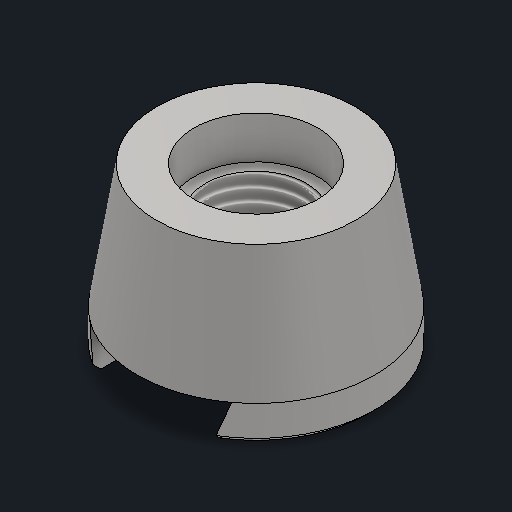
# Autodesk Inventor part: 0.375 Shaft Dovetail
Saved by Autodesk Inventor 2025.1 (Build 291241020, 241B)
## iProperties
Created: 2025-05-15
Part Number: 0.375 Shaft Dovetail
Material: Stainless Steel
Document SubType Name: Modeling
Designer: Joshua Eah
Density: 8 g/cm^3
Appearance: Semi-Polished
Author: Joshua Eah
Autodesk Inventor part; units mm, degrees
ref_plane "YZ Plane" through (0, 0, 0) normal (1, 0, 0) x (0, 1, 0)
sketch "Sketch1" plane through (0, 0, 0) normal (0, 1, 0) x (-1, 0, 0)
  circle A0 centre (0, 0) radius 4.9911
  dimension "d0" = 9.9822
  constraints: 1 centre point, 1 coincident
  measures "d0" diameter of A0
extrude "Extrusion1" add sketch "Sketch1" along normal blind 1.524
sketch "Sketch2" plane through (0, 1.524, 0) normal (0, 1, 0) x (1, 0, 0)
  point P0 (0, 0)
ref_plane "Work Plane1" through (0, 6.731, 0) normal (0, -1, 0) x (1, 0, 0)
sketch "Sketch3" plane through (0, 6.731, 0) normal (0, -1, 0) x (1, 0, 0)
  circle A0 centre (0, 0) radius 4.1593
  circle A1 centre (0, 0) radius 2.6035
  dimension "d4" = 8.3185
  dimension "d9" = 5.207
  constraints: 2 centre point, 2 coincident
  measures "d4" diameter of A0
  measures "d9" diameter of A1
loft "Loft1" add profiles "Sketch3" section 1 edges at (4.9911, 1.524, 0) contours A0 | A1
hole "Hole1" at (0, 6.731, 0) direction (0, -1, 0) diameter 4.2418 end through all thread size "10-48 UNS" class "2B" standard "ANSI Unified Screw Threads"
extrude "Extrusion3" cut sketch "Sketch3" along normal blind 1.778 contours A1
ref_plane "Work Plane2" through (0, 0, -4.9911) normal (0, 0, 1) x (1, 0, 0)
chamfer "Chamfer1" distance 0.254 angle 45 1 edges at (4.9911, 0, 0)
sketch "Sketch4" plane through (0, 0, -4.9911) normal (0, 0, 1) x (1, 0, 0)
  line L0 (4.9911, 1.524) -> (-4.9911, 1.524) projected
  line L1 (0, 1.524) -> (0, 0)
  line L2 (2.5082, 1.524) -> (-2.5083, 1.524)
  line L3 (-2.5083, 1.524) -> (-2.5083, 0)
  line L4 (-2.5083, 0) -> (2.5082, 0)
  line L5 (2.5082, 0) -> (2.5082, 1.524)
  line L6 (2.5082, 1.524) -> (-2.5083, 0) construction
  line L7 (-2.5083, 1.524) -> (2.5082, 0) construction
  line L8 (2.9845, 1.524) -> (-2.9845, 1.524)
  line L9 (-2.9845, 1.524) -> (-2.9845, 0)
  line L10 (-2.9845, 0) -> (2.9845, 0)
  line L11 (2.9845, 0) -> (2.9845, 1.524)
  line L12 (2.9845, 1.524) -> (-2.9845, 0) construction
  line L13 (-2.9845, 1.524) -> (2.9845, 0) construction
  line L14 (2.9845, 1.524) -> (2.5082, 0)
  line L15 (-2.9845, 1.524) -> (-2.5083, 0)
  point P0 (4.9911, 0)
  point P1 (-4.9911, 0)
  point P2 (0, 0.762)
  dimension "d23" = 5.0165
  dimension "d24" = 5.969
  constraints: 30 end point, 6 midpoint, 4 parallel, 2 horizontal, 2 perpendicular
  measures "d23" distance of L4.end L3.end
  measures "d24" distance of L10.end L9.end
extrude "Extrusion4" cut sketch "Sketch4" along normal through all contours L14 L5 L0 | L5 L4 L1 L0 | L1 L4 L3 L0 | L3 L15 L0
body "Solid1"
